Autodesk Inventor part; units mm, degrees
(part 6 of 6)
sketch "Sketch4" plane through (0, 0, 0) normal (0, 0, -1) x (-1, 0, 0)
  line L0 (64.8722, 81.696) -> (64.8722, 215.6959) projected
  line L1 (-12.6282, 191.1959) -> (-197.1645, 191.1959) projected
  line L2 (-224.6643, 218.6959) -> (-272.1277, 218.6959) projected
  line L3 (-275.1277, 215.6959) -> (-275.1277, 81.696) projected
  circle A0 centre (-267.6277, 209.6959) radius 3
  circle A1 centre (-248.6277, 199.1959) radius 9
  circle A2 centre (-248.6277, 171.1959) radius 9
  circle A3 centre (-267.6277, 148.6959) radius 3
  circle A4 centre (-225.1277, 202.1959) radius 6
  line L4 (-275.1277, 148.6959) -> (64.8722, 148.6959) construction
  circle A5 centre (-225.1277, 185.295) radius 2.75
  circle A6 centre (-248.1277, 148.6959) radius 6
  circle A7 centre (-209.6277, 170.4137) radius 4.5
  circle A8 centre (-267.6277, 87.696) radius 3
  circle A9 centre (-248.6277, 98.196) radius 9
  circle A10 centre (-248.6277, 126.196) radius 9
  circle A11 centre (-225.1277, 95.196) radius 6
  circle A12 centre (-225.1277, 112.0968) radius 2.75
  circle A13 centre (-209.6277, 126.9781) radius 4.5
  line L5 (-234.1277, 133.6959) -> (-216.1277, 133.6959)
  line L6 (-212.1277, 137.6959) -> (-212.1277, 159.6959)
  line L7 (-216.1277, 163.6959) -> (-234.1277, 163.6959)
  line L8 (-238.1277, 159.6959) -> (-238.1277, 137.6959)
  line L9 (-238.1277, 133.6959) -> (-212.1277, 163.6959) construction
  line L10 (-212.1277, 133.6959) -> (-238.1277, 163.6959) construction
  arc A14 (-234.1277, 163.6959) -> (-238.1277, 159.6959) centre (-234.1277, 159.6959) ccw
  arc A15 (-212.1277, 159.6959) -> (-216.1277, 163.6959) centre (-216.1277, 159.6959) ccw
  arc A16 (-216.1277, 133.6959) -> (-212.1277, 137.6959) centre (-216.1277, 137.6959) ccw
  arc A17 (-238.1277, 137.6959) -> (-234.1277, 133.6959) centre (-234.1277, 137.6959) ccw
  line L11 (-195.6277, 118.1959) -> (-121.6277, 118.1959)
  line L12 (-115.6277, 124.1959) -> (-115.6277, 173.1959)
  line L13 (-121.6277, 179.1959) -> (-195.6277, 179.1959)
  line L14 (-201.6277, 173.1959) -> (-201.6277, 124.1959)
  line L15 (-201.6277, 118.1959) -> (-115.6277, 179.1959) construction
  line L16 (-115.6277, 118.1959) -> (-201.6277, 179.1959) construction
  arc A18 (-195.6277, 179.1959) -> (-201.6277, 173.1959) centre (-195.6277, 173.1959) ccw
  arc A19 (-115.6277, 173.1959) -> (-121.6277, 179.1959) centre (-121.6277, 173.1959) ccw
  arc A20 (-121.6277, 118.1959) -> (-115.6277, 124.1959) centre (-121.6277, 124.1959) ccw
  arc A21 (-201.6277, 124.1959) -> (-195.6277, 118.1959) centre (-195.6277, 124.1959) ccw
  line L17 (-107.4278, 140.1959) -> (-102.8278, 140.1959)
  line L18 (-98.8278, 144.1959) -> (-98.8278, 153.1959)
  line L19 (-102.8278, 157.1959) -> (-107.4278, 157.1959)
  line L20 (-111.4278, 153.1959) -> (-111.4278, 144.1959)
  line L21 (-111.4278, 140.1959) -> (-98.8278, 157.1959) construction
  line L22 (-98.8278, 140.1959) -> (-111.4278, 157.1959) construction
  arc A22 (-107.4278, 157.1959) -> (-111.4278, 153.1959) centre (-107.4278, 153.1959) ccw
  arc A23 (-98.8278, 153.1959) -> (-102.8278, 157.1959) centre (-102.8278, 153.1959) ccw
  arc A24 (-102.8278, 140.1959) -> (-98.8278, 144.1959) centre (-102.8278, 144.1959) ccw
  arc A25 (-111.4278, 144.1959) -> (-107.4278, 140.1959) centre (-107.4278, 144.1959) ccw
  line L23 (-107.4278, 162.1959) -> (-102.8278, 162.1959)
  line L24 (-98.8278, 166.1959) -> (-98.8278, 175.1959)
  line L25 (-102.8278, 179.1959) -> (-107.4278, 179.1959)
  line L26 (-111.4278, 175.1959) -> (-111.4278, 166.1959)
  line L27 (-111.4278, 162.1959) -> (-98.8278, 179.1959) construction
  line L28 (-98.8278, 162.1959) -> (-111.4278, 179.1959) construction
  arc A26 (-107.4278, 179.1959) -> (-111.4278, 175.1959) centre (-107.4278, 175.1959) ccw
  arc A27 (-98.8278, 175.1959) -> (-102.8278, 179.1959) centre (-102.8278, 175.1959) ccw
  arc A28 (-102.8278, 162.1959) -> (-98.8278, 166.1959) centre (-102.8278, 166.1959) ccw
  arc A29 (-111.4278, 166.1959) -> (-107.4278, 162.1959) centre (-107.4278, 166.1959) ccw
  line L29 (-107.4278, 118.1959) -> (-102.8278, 118.1959)
  line L30 (-98.8278, 122.1959) -> (-98.8278, 131.1959)
  line L31 (-102.8278, 135.1959) -> (-107.4278, 135.1959)
  line L32 (-111.4278, 131.1959) -> (-111.4278, 122.1959)
  line L33 (-111.4278, 118.1959) -> (-98.8278, 135.1959) construction
  line L34 (-98.8278, 118.1959) -> (-111.4278, 135.1959) construction
  arc A30 (-107.4278, 135.1959) -> (-111.4278, 131.1959) centre (-107.4278, 131.1959) ccw
  arc A31 (-98.8278, 131.1959) -> (-102.8278, 135.1959) centre (-102.8278, 131.1959) ccw
  arc A32 (-102.8278, 118.1959) -> (-98.8278, 122.1959) centre (-102.8278, 122.1959) ccw
  arc A33 (-111.4278, 122.1959) -> (-107.4278, 118.1959) centre (-107.4278, 122.1959) ccw
  line L35 (-107.4278, 140.1959) -> (-102.8278, 140.1959)
  line L36 (-98.8278, 144.1959) -> (-98.8278, 153.1959)
  line L37 (-102.8278, 157.1959) -> (-107.4278, 157.1959)
  line L38 (-111.4278, 153.1959) -> (-111.4278, 144.1959)
  line L39 (-111.4278, 140.1959) -> (-98.8278, 157.1959) construction
  line L40 (-98.8278, 140.1959) -> (-111.4278, 157.1959) construction
  arc A34 (-107.4278, 157.1959) -> (-111.4278, 153.1959) centre (-107.4278, 153.1959) ccw
  arc A35 (-98.8278, 153.1959) -> (-102.8278, 157.1959) centre (-102.8278, 153.1959) ccw
  arc A36 (-102.8278, 140.1959) -> (-98.8278, 144.1959) centre (-102.8278, 144.1959) ccw
  arc A37 (-111.4278, 144.1959) -> (-107.4278, 140.1959) centre (-107.4278, 144.1959) ccw
  line L41 (-91.3278, 118.1959) -> (-61.8278, 118.1959)
  line L42 (-57.8278, 122.1959) -> (-57.8278, 175.1959)
  line L43 (-61.8278, 179.1959) -> (-84.3278, 179.1959)
  line L44 (-95.3278, 168.1959) -> (-95.3278, 122.1959)
  line L45 (-95.3278, 118.1959) -> (-57.8278, 179.1959) construction
  line L46 (-57.8278, 118.1959) -> (-95.3278, 179.1959) construction
  line L47 (-84.3278, 179.1959) -> (-95.3278, 168.1959)
  arc A38 (-57.8278, 175.1959) -> (-61.8278, 179.1959) centre (-61.8278, 175.1959) ccw
  arc A39 (-61.8278, 118.1959) -> (-57.8278, 122.1959) centre (-61.8278, 122.1959) ccw
  arc A40 (-95.3278, 122.1959) -> (-91.3278, 118.1959) centre (-91.3278, 122.1959) ccw
  line L48 (-52.6278, 143.6959) -> (-51.8278, 143.6959)
  line L49 (-49.3278, 146.1959) -> (-49.3278, 151.1959)
  line L50 (-51.8278, 153.6959) -> (-52.6278, 153.6959)
  line L51 (-55.1278, 151.1959) -> (-55.1278, 146.1959)
  line L52 (-55.1278, 143.6959) -> (-49.3278, 153.6959) construction
  line L53 (-49.3278, 143.6959) -> (-55.1278, 153.6959) construction
  arc A41 (-52.6278, 153.6959) -> (-55.1278, 151.1959) centre (-52.6278, 151.1959) ccw
  arc A42 (-49.3278, 151.1959) -> (-51.8278, 153.6959) centre (-51.8278, 151.1959) ccw
  arc A43 (-51.8278, 143.6959) -> (-49.3278, 146.1959) centre (-51.8278, 146.1959) ccw
  arc A44 (-55.1278, 146.1959) -> (-52.6278, 143.6959) centre (-52.6278, 146.1959) ccw
  line L54 (-275.1277, 161.3959) -> (64.8722, 161.3959) construction
  line L55 (-52.6278, 156.3959) -> (-51.8278, 156.3959)
  line L56 (-49.3278, 158.8959) -> (-49.3278, 163.8959)
  line L57 (-51.8278, 166.3959) -> (-52.6278, 166.3959)
  line L58 (-55.1278, 163.8959) -> (-55.1278, 158.8959)
  line L59 (-55.1278, 156.3959) -> (-49.3278, 166.3959) construction
  line L60 (-49.3278, 156.3959) -> (-55.1278, 166.3959) construction
  arc A45 (-52.6278, 166.3959) -> (-55.1278, 163.8959) centre (-52.6278, 163.8959) ccw
  arc A46 (-49.3278, 163.8959) -> (-51.8278, 166.3959) centre (-51.8278, 163.8959) ccw
  arc A47 (-51.8278, 156.3959) -> (-49.3278, 158.8959) centre (-51.8278, 158.8959) ccw
  arc A48 (-55.1278, 158.8959) -> (-52.6278, 156.3959) centre (-52.6278, 158.8959) ccw
  line L61 (-275.1277, 174.0959) -> (64.8722, 174.0959) construction
  line L62 (-52.6278, 169.0959) -> (-51.8278, 169.0959)
  line L63 (-49.3278, 171.5959) -> (-49.3278, 176.5959)
  line L64 (-51.8278, 179.0959) -> (-52.6278, 179.0959)
  line L65 (-55.1278, 176.5959) -> (-55.1278, 171.5959)
  line L66 (-55.1278, 169.0959) -> (-49.3278, 179.0959) construction
  line L67 (-49.3278, 169.0959) -> (-55.1278, 179.0959) construction
  arc A49 (-52.6278, 179.0959) -> (-55.1278, 176.5959) centre (-52.6278, 176.5959) ccw
  arc A50 (-49.3278, 176.5959) -> (-51.8278, 179.0959) centre (-51.8278, 176.5959) ccw
  arc A51 (-51.8278, 169.0959) -> (-49.3278, 171.5959) centre (-51.8278, 171.5959) ccw
  arc A52 (-55.1278, 171.5959) -> (-52.6278, 169.0959) centre (-52.6278, 171.5959) ccw
  line L68 (-275.1277, 135.9959) -> (64.8722, 135.9959) construction
  line L69 (-52.6278, 130.9959) -> (-51.8278, 130.9959)
  line L70 (-49.3278, 133.4959) -> (-49.3278, 138.4959)
  line L71 (-51.8278, 140.9959) -> (-52.6278, 140.9959)
  line L72 (-55.1278, 138.4959) -> (-55.1278, 133.4959)
  line L73 (-55.1278, 130.9959) -> (-49.3278, 140.9959) construction
  line L74 (-49.3278, 130.9959) -> (-55.1278, 140.9959) construction
  arc A53 (-52.6278, 140.9959) -> (-55.1278, 138.4959) centre (-52.6278, 138.4959) ccw
  arc A54 (-49.3278, 138.4959) -> (-51.8278, 140.9959) centre (-51.8278, 138.4959) ccw
  arc A55 (-51.8278, 130.9959) -> (-49.3278, 133.4959) centre (-51.8278, 133.4959) ccw
  arc A56 (-55.1278, 133.4959) -> (-52.6278, 130.9959) centre (-52.6278, 133.4959) ccw
  line L75 (-275.1277, 148.6959) -> (64.8722, 148.6959) construction
  line L76 (-52.6278, 143.6959) -> (-51.8278, 143.6959)
  line L77 (-49.3278, 146.1959) -> (-49.3278, 151.1959)
  line L78 (-51.8278, 153.6959) -> (-52.6278, 153.6959)
  line L79 (-55.1278, 151.1959) -> (-55.1278, 146.1959)
  line L80 (-55.1278, 143.6959) -> (-49.3278, 153.6959) construction
  line L81 (-49.3278, 143.6959) -> (-55.1278, 153.6959) construction
  arc A57 (-52.6278, 153.6959) -> (-55.1278, 151.1959) centre (-52.6278, 151.1959) ccw
  arc A58 (-49.3278, 151.1959) -> (-51.8278, 153.6959) centre (-51.8278, 151.1959) ccw
  arc A59 (-51.8278, 143.6959) -> (-49.3278, 146.1959) centre (-51.8278, 146.1959) ccw
  arc A60 (-55.1278, 146.1959) -> (-52.6278, 143.6959) centre (-52.6278, 146.1959) ccw
  line L82 (-275.1277, 161.3959) -> (64.8722, 161.3959) construction
  line L83 (-52.6278, 156.3959) -> (-51.8278, 156.3959)
  line L84 (-49.3278, 158.8959) -> (-49.3278, 163.8959)
  line L85 (-51.8278, 166.3959) -> (-52.6278, 166.3959)
  line L86 (-55.1278, 163.8959) -> (-55.1278, 158.8959)
  line L87 (-55.1278, 156.3959) -> (-49.3278, 166.3959) construction
  line L88 (-49.3278, 156.3959) -> (-55.1278, 166.3959) construction
  arc A61 (-52.6278, 166.3959) -> (-55.1278, 163.8959) centre (-52.6278, 163.8959) ccw
  arc A62 (-49.3278, 163.8959) -> (-51.8278, 166.3959) centre (-51.8278, 163.8959) ccw
  arc A63 (-51.8278, 156.3959) -> (-49.3278, 158.8959) centre (-51.8278, 158.8959) ccw
  arc A64 (-55.1278, 158.8959) -> (-52.6278, 156.3959) centre (-52.6278, 158.8959) ccw
  line L89 (-275.1277, 123.2959) -> (64.8722, 123.2959) construction
  line L90 (-52.6278, 118.2959) -> (-51.8278, 118.2959)
  line L91 (-49.3278, 120.7959) -> (-49.3278, 125.7959)
  line L92 (-51.8278, 128.2959) -> (-52.6278, 128.2959)
  line L93 (-55.1278, 125.7959) -> (-55.1278, 120.7959)
  line L94 (-55.1278, 118.2959) -> (-49.3278, 128.2959) construction
  line L95 (-49.3278, 118.2959) -> (-55.1278, 128.2959) construction
  arc A65 (-52.6278, 128.2959) -> (-55.1278, 125.7959) centre (-52.6278, 125.7959) ccw
  arc A66 (-49.3278, 125.7959) -> (-51.8278, 128.2959) centre (-51.8278, 125.7959) ccw
  arc A67 (-51.8278, 118.2959) -> (-49.3278, 120.7959) centre (-51.8278, 120.7959) ccw
  arc A68 (-55.1278, 120.7959) -> (-52.6278, 118.2959) centre (-52.6278, 120.7959) ccw
  line L96 (-275.1277, 135.9959) -> (64.8722, 135.9959) construction
  line L97 (-52.6278, 130.9959) -> (-51.8278, 130.9959)
  line L98 (-49.3278, 133.4959) -> (-49.3278, 138.4959)
  line L99 (-51.8278, 140.9959) -> (-52.6278, 140.9959)
  line L100 (-55.1278, 138.4959) -> (-55.1278, 133.4959)
  line L101 (-55.1278, 130.9959) -> (-49.3278, 140.9959) construction
  line L102 (-49.3278, 130.9959) -> (-55.1278, 140.9959) construction
  arc A69 (-52.6278, 140.9959) -> (-55.1278, 138.4959) centre (-52.6278, 138.4959) ccw
  arc A70 (-49.3278, 138.4959) -> (-51.8278, 140.9959) centre (-51.8278, 138.4959) ccw
  arc A71 (-51.8278, 130.9959) -> (-49.3278, 133.4959) centre (-51.8278, 133.4959) ccw
  arc A72 (-55.1278, 133.4959) -> (-52.6278, 130.9959) centre (-52.6278, 133.4959) ccw
  line L103 (-275.1277, 148.6959) -> (64.8722, 148.6959) construction
  line L104 (-52.6278, 143.6959) -> (-51.8278, 143.6959)
  line L105 (-49.3278, 146.1959) -> (-49.3278, 151.1959)
  line L106 (-51.8278, 153.6959) -> (-52.6278, 153.6959)
  line L107 (-55.1278, 151.1959) -> (-55.1278, 146.1959)
  line L108 (-55.1278, 143.6959) -> (-49.3278, 153.6959) construction
  line L109 (-49.3278, 143.6959) -> (-55.1278, 153.6959) construction
  arc A73 (-52.6278, 153.6959) -> (-55.1278, 151.1959) centre (-52.6278, 151.1959) ccw
  arc A74 (-49.3278, 151.1959) -> (-51.8278, 153.6959) centre (-51.8278, 151.1959) ccw
  arc A75 (-51.8278, 143.6959) -> (-49.3278, 146.1959) centre (-51.8278, 146.1959) ccw
  arc A76 (-55.1278, 146.1959) -> (-52.6278, 143.6959) centre (-52.6278, 146.1959) ccw
  line L110 (-12.7278, 118.1959) -> (-42.2278, 118.1959)
  line L111 (-46.2278, 122.1959) -> (-46.2278, 175.1959)
  line L112 (-42.2278, 179.1959) -> (-12.7278, 179.1959)
  line L113 (-8.7278, 175.1959) -> (-8.7278, 122.1959)
  line L114 (-8.7278, 118.1959) -> (-46.2278, 179.1959) construction
  line L115 (-46.2278, 118.1959) -> (-8.7278, 179.1959) construction
  arc A77 (-42.2278, 179.1959) -> (-46.2278, 175.1959) centre (-42.2278, 175.1959) ccw
  arc A78 (-8.7278, 175.1959) -> (-12.7278, 179.1959) centre (-12.7278, 175.1959) ccw
  arc A79 (-46.2278, 122.1959) -> (-42.2278, 118.1959) centre (-42.2278, 122.1959) ccw
  arc A80 (-12.7278, 118.1959) -> (-8.7278, 122.1959) centre (-12.7278, 122.1959) ccw
  line L116 (5.7722, 133.6959) -> (23.7722, 133.6959)
  line L117 (27.7722, 137.6959) -> (27.7722, 159.6959)
  line L118 (23.7722, 163.6959) -> (5.7722, 163.6959)
  line L119 (1.7722, 159.6959) -> (1.7722, 137.6959)
  line L120 (1.7722, 133.6959) -> (27.7722, 163.6959) construction
  line L121 (27.7722, 133.6959) -> (1.7722, 163.6959) construction
  arc A81 (5.7722, 163.6959) -> (1.7722, 159.6959) centre (5.7722, 159.6959) ccw
  arc A82 (27.7722, 159.6959) -> (23.7722, 163.6959) centre (23.7722, 159.6959) ccw
  arc A83 (23.7722, 133.6959) -> (27.7722, 137.6959) centre (23.7722, 137.6959) ccw
  arc A84 (1.7722, 137.6959) -> (5.7722, 133.6959) centre (5.7722, 137.6959) ccw
  circle A85 centre (-112.1277, 185.1959) radius 2.1
  circle A86 centre (-98.1277, 185.1959) radius 2.1
  circle A87 centre (-84.1277, 185.1959) radius 2.1
  circle A88 centre (-70.1277, 185.1959) radius 2.1
  circle A89 centre (-56.1277, 185.1959) radius 2.1
  circle A90 centre (-42.1277, 185.1959) radius 2.1
  circle A91 centre (-28.1277, 185.1959) radius 2.1
  circle A92 centre (-14.1277, 185.1959) radius 2.1
  circle A93 centre (-112.1277, 112.1959) radius 2.1
  circle A94 centre (-98.1277, 112.1959) radius 2.1
  circle A95 centre (-84.1277, 112.1959) radius 2.1
  circle A96 centre (-70.1277, 112.1959) radius 2.1
  circle A97 centre (-56.1277, 112.1959) radius 2.1
  circle A98 centre (-42.1277, 112.1959) radius 2.1
  circle A99 centre (-28.1277, 112.1959) radius 2.1
  circle A100 centre (-14.1277, 112.1959) radius 2.1
  line L122 (61.8722, 218.6959) -> (14.8718, 218.6959) projected
  circle A101 centre (-0.7278, 170.3959) radius 4.5
  circle A102 centre (37.7722, 171.1959) radius 9
  circle A103 centre (14.8723, 185.1959) radius 2.75
  circle A104 centre (14.8723, 202.1959) radius 6
  circle A105 centre (37.7722, 199.1959) radius 9
  circle A106 centre (-0.7278, 126.9959) radius 4.5
  circle A107 centre (37.7722, 126.1959) radius 9
  circle A108 centre (14.8723, 112.1959) radius 2.75
  circle A109 centre (14.8723, 95.196) radius 6
  circle A110 centre (37.7722, 98.196) radius 9
  line L123 (14.8739, 78.696) -> (61.8722, 78.696) projected
  circle A111 centre (57.3722, 87.696) radius 3
  circle A112 centre (57.3722, 96.196) radius 2
  circle A113 centre (57.3722, 209.6959) radius 3
  circle A114 centre (57.3722, 201.1959) radius 2
  circle A115 centre (53.8723, 185.1959) radius 6
  circle A116 centre (53.8723, 153.1959) radius 6
  point P0 (0, 0)
  point P1 (-225.1277, 148.6959)
  point P2 (-158.6277, 148.6959)
  point P3 (-105.1278, 148.6959)
  point P4 (-105.1278, 170.6959)
  point P5 (-105.1278, 126.6959)
  point P6 (-105.1278, 148.6959)
  point P7 (-76.5778, 148.6959)
  point P8 (-52.2278, 148.6959)
  point P9 (-248.1277, 161.3959)
  point P10 (-225.1277, 161.3959)
  point P11 (-158.6277, 161.3959)
  point P12 (-105.1278, 161.3959)
  point P13 (-76.5778, 161.3959)
  point P14 (-52.2278, 161.3959)
  point P15 (-248.1277, 174.0959)
  point P16 (-225.1277, 174.0959)
  point P17 (-158.6277, 174.0959)
  point P18 (-105.1278, 174.0959)
  point P19 (-76.5778, 174.0959)
  point P20 (-52.2278, 174.0959)
  point P21 (-248.1277, 135.9959)
  point P22 (-225.1277, 135.9959)
  point P23 (-158.6277, 135.9959)
  point P24 (-105.1278, 135.9959)
  point P25 (-76.5778, 135.9959)
  point P26 (-52.2278, 135.9959)
  point P27 (-225.1277, 148.6959)
  point P28 (-158.6277, 148.6959)
  point P29 (-105.1278, 148.6959)
  point P30 (-76.5778, 148.6959)
  point P31 (-52.2278, 148.6959)
  point P32 (-248.1277, 161.3959)
  point P33 (-225.1277, 161.3959)
  point P34 (-158.6277, 161.3959)
  point P35 (-105.1278, 161.3959)
  point P36 (-76.5778, 161.3959)
  point P37 (-52.2278, 161.3959)
  point P38 (-248.1277, 123.2959)
  point P39 (-225.1277, 123.2959)
  point P40 (-158.6277, 123.2959)
  point P41 (-105.1278, 123.2959)
  point P42 (-76.5778, 123.2959)
  point P43 (-52.2278, 123.2959)
  point P44 (-248.1277, 135.9959)
  point P45 (-225.1277, 135.9959)
  point P46 (-158.6277, 135.9959)
  point P47 (-105.1278, 135.9959)
  point P48 (-76.5778, 135.9959)
  point P49 (-52.2278, 135.9959)
  point P50 (-225.1277, 148.6959)
  point P51 (-158.6277, 148.6959)
  point P52 (-105.1278, 148.6959)
  point P53 (-76.5778, 148.6959)
  point P54 (-52.2278, 148.6959)
  point P55 (-27.4778, 148.6959)
  point P56 (14.7722, 148.6959)
  dimension "d2" = 6
  dimension "d3" = 7.5
  dimension "d4" = 9
  dimension "d5" = 18
  dimension "d6" = 19
  dimension "d7" = 10.5
  dimension "d8" = 18
  dimension "d9" = 28
  dimension "d10" = 26.5
  dimension "d11" = 6
  dimension "d12" = 7.5
  dimension "d13" = 69.9999
  dimension "d14" = 12
  dimension "d15" = 23.5
  dimension "d16" = 16.5
  dimension "d17" = 5.5
  dimension "d18" = 16.9008
  dimension "d19" = 50
  dimension "d20" = 12
  dimension "d21" = 19.5
  dimension "d22" = 9
  dimension "d23" = 39
  dimension "d24" = 20.7822
  dimension "d25" = 26
  dimension "d26" = 30
  dimension "d27" = 4
  dimension "d28" = 4
  dimension "d31" = 86
  dimension "d32" = 10.5
  dimension "d33" = 37
  dimension "d34" = 61
  dimension "d35" = 6
  dimension "d36" = 17
  dimension "d37" = 12.6
  dimension "d38" = 4
  dimension "d41" = 22
  dimension "d44" = 22
  dimension "d47" = 37.5
  dimension "d48" = 3.5
  dimension "d49" = 61
  dimension "d50" = 11
  dimension "d51" = 11
  dimension "d52" = 4
  dimension "d53" = 4
  dimension "d54" = 5.8
  dimension "d55" = 10
  dimension "d56" = 2.7
  dimension "d57" = 2.5
  dimension "d60" = 12.7
  dimension "d63" = 12.7
  dimension "d66" = 37.5
  dimension "d67" = 4
  dimension "d68" = 3.1
  dimension "d69" = 26
  dimension "d70" = 30
  dimension "d71" = 10.5
  dimension "d72" = 4
  dimension "d73" = 6
  dimension "d74" = 4.2
  dimension "d75" = 3.5
  dimension "d78" = 14
  dimension "d83" = 6.7
  dimension "d84" = 9
  dimension "d85" = 8
  constraints: 234 end point, 184 point on line, 142 point on circle, 117 centre point, 54 tangent, 39 midpoint, 21 symmetric about line, 18 equal radius, 14 parallel, 8 horizontal, 8 perpendicular, 4 vertical, 1 collinear, 405 other
  measures "d2" diameter of A0
  measures "d3" distance from line of L3 A0.centre
  measures "d4" distance from line of L2 A0.centre
  measures "d5" diameter of A1
  measures "d6" horizontal distance of A1.centre A0.centre
  measures "d7" vertical distance of A1.centre A0.centre
  measures "d8" diameter of A2
  measures "d9" distance of A1.centre A2.centre
  measures "d10" distance from line of L3 A2.centre
  measures "d11" diameter of A3
  measures "d12" distance from line of L3 A3.centre
  measures "d13" distance from line of L2 A3.centre
  measures "d14" diameter of A4
  measures "d15" horizontal distance of A1.centre A4.centre
  measures "d16" distance from line of L2 A4.centre
  measures "d17" diameter of A5
  measures "d18" distance of A4.centre A5.centre
  measures "d19" distance from line of L3 A5.centre
  measures "d20" diameter of A6
  measures "d21" distance of A3.centre A6.centre
  measures "d22" diameter of A7
  measures "d23" horizontal distance of A2.centre A7.centre
  measures "d24" distance from line of L1 A7.centre
  measures "d25" distance between parallel lines of L6 L8
  measures "d26" distance of L10.start L9.end
  measures "d27" radius of A14
  measures "d28" radius of A17
  measures "d31" distance between parallel lines of L12 L14
  measures "d32" distance between parallel lines of L6 L14
  measures "d33" distance between parallel lines of L3 L8
  measures "d34" distance between parallel lines of L11 L13
  measures "d35" radius of A18
  measures "d36" distance between parallel lines of L17 L19
  measures "d37" distance between parallel lines of L20 L18
  measures "d38" radius of A22
  measures "d41" distance of L17.start L23.start
  measures "d44" distance of L17.start L29.start
  measures "d47" distance between parallel lines of L44 L42
  measures "d48" distance between parallel lines of L24 L44
  measures "d49" distance between parallel lines of L41 L43
  measures "d50" distance of L43.end L46.end
  measures "d51" distance of L44.start L46.end
  measures "d52" radius of A38
  measures "d53" radius of A39
  measures "d54" distance of L52.end L53.end
  measures "d55" distance of L53.end L52.start
  measures "d56" distance between parallel lines of L42 L51
  measures "d57" radius of A41
  measures "d60" distance of L4.start L54.start
  measures "d63" distance of L4.start L68.start
  measures "d66" distance of L114.end L115.end
  measures "d67" radius of A77
  measures "d68" distance between parallel lines of L70 L111
  measures "d69" distance of L120.end L121.end
  measures "d70" distance of L121.end L120.start
  measures "d71" distance between parallel lines of L113 L119
  measures "d72" radius of A81
  measures "d73" distance from line of L1 A85.centre
  measures "d74" diameter of A85
  measures "d75" distance from line of L12 A85.centre
  measures "d78" distance of A85.centre A86.centre
  measures "d83" distance from line of L118 A101.centre
  measures "d84" diameter of A101
  measures "d85" distance from line of L113 A101.centre
extrude "Extrusion2" cut sketch "Sketch4" against normal through all contours A0 | A1 | A2 | A3 | A4 | A5 | A6 | A7 | A8 | A9 | A10 | A11 | A12 | A13 | A17 L8 A14 L7 A15 L6 A16 L5 | A21 L14 A18 L13 A19 L12 A20 L11 | A25 L20 A22 L19 A23 L18 A24 L17 | A29 L26 A26 L25 A27 L24 A28 L23 | A33 L32 A30 L31 A31 L30 A32 L29 | A40 L44 L47 L43 A38 L42 A39 L41 | A44 L51 A41 L50 A42 L49 A43 L48 | A48 L58 A45 L57 A46 L56 A47 L55 | A52 L65 A49 L64 A50 L63 A51 L62 | A56 L72 A53 L71 A54 L70 A55 L69 | A68 L93 A65 L92 A66 L91 A67 L90 | L110 A79 L111 A77 L112 A78 L113 A80 | A84 L119 A81 L118 A82 L117 A83 L116 | A85 | A86 | A87 | A88 | A89 | A90 | A91 | A92 | A93 | A94 | A95 | A96 | A97 | A98 | A99 | A100 | A101 | A102 | A103 | A104 | A105 | A106 | A107 | A108 | A109 | A110 | A113 | A114 | A115 | A116
ref_plane "Work Plane1" through (105.1278, 81.696, 0) normal (-1, 0, 0) x (0, 0, 1)
ref_plane "Work Plane2" through (224.6664, 148.6959, 0) normal (0, -1, 0) x (1, 0, 0)
equation "\"d51\" = d50"
body "Solid1"
